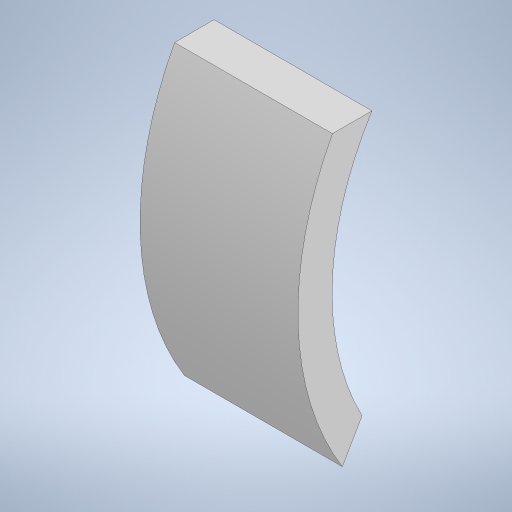
# Autodesk Inventor part: Gripper
Saved by Autodesk Inventor 2024 (Build 280153000, 153)
## iProperties
Created: 2024-01-03
Part Number: Gripper
Material: Generic
Document SubType Name: Modeling
Designer: mrizw
Density: 1 g/cm^3
Appearance: Default
Author: mrizw
Autodesk Inventor part; units mm, degrees
ref_plane "YZ Plane" through (0, 0, 0) normal (1, 0, 0) x (0, 1, 0)
ref_plane "XZ Plane" through (0, 0, 0) normal (0, 1, 0) x (-1, 0, 0)
ref_plane "XY Plane" through (0, 0, 0) normal (0, 0, 1) x (1, 0, 0)
sketch "Sketch5" plane through (0, 0, 0) normal (1, 0, 0) x (0, 1, 0)
  arc A0 (0, -5) -> (-70, -5) centre (-35, -65.6218) ccw
  line L0 (0, -5) -> (-70, -5) construction
  line L1 (0, -5) -> (70, -5) construction
  point P0 (0, 0)
  dimension "d4" = 5
  dimension "d5" = 70
  dimension "d6" = 180
  dimension "d7" = 70
  constraints: 4 end point, 2 point on circle, 1 centre point, 1 collinear, 1 horizontal
  measures "d4" distance of point (0, 0) L0.start
  measures "d5" distance of L0.start L0.end
  measures "d6" angle of L0 L1
  measures "d7" radius of A0
sketch "Sketch7" plane through (0, 0, 0) normal (0, 1, 0) x (-1, 0, 0)
  line L0 (20, 0) -> (-20, 0)
  line L1 (-20, 0) -> (-20, -10)
  line L2 (-20, -10) -> (20, -10)
  line L3 (20, -10) -> (20, 0)
  point P0 (0, 0)
  dimension "d13" = 40
  dimension "d14" = 10
  constraints: 8 end point, 2 parallel, 1 horizontal, 1 perpendicular
  measures "d13" distance of L2.end L1.end
  measures "d14" distance of L1.end L0.end
sweep "Sweep1" add profiles "Sketch7" path "Sketch5"
body "Solid1"
